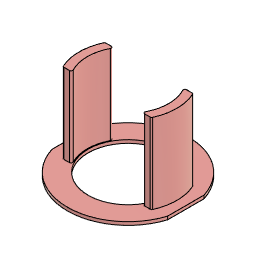
pelican TSA key retainer v1 (Autodesk Fusion 360 design; units mm, degrees)
Autodesk Fusion 360 part; units mm, degrees
note: some values were not read from the file. Set by a fixed rule: which sketch regions a step uses.
sketch "Sketch1" plane through (0, 0, 0) normal (0, 0, 1) x (1, 0, 0)
  circle A0 centre (0, 0) radius 6.3
  circle A1 centre (0, 0) radius 7.6
  line L0 (0, 7.6) -> (0, -7.6) construction
  circle A2 centre (0, 0) radius 3.25
  line L1 (-3.25, 0) -> (-3.25, -3.35)
  line L2 (-3.25, -3.35) -> (3.25, -3.35)
  line L3 (3.25, 0) -> (3.25, -3.35)
  circle A3 centre (0, 0) radius 5
  dimension "d1" = 12.6
  dimension "d2" = 15.2
  dimension "d3" = 6.5
  dimension "d4" = 3.35
  dimension "d15" = 10
  constraint coincident A0.centre A1.centre
  constraint coincident A1 L0.start
  constraint coincident A1 L0.end
  constraint vertical L0
  constraint coincident L0 A0.centre
  constraint coincident A2 L1.start
  constraint tangent A2 L1
  constraint parallel L0 L1
  constraint perpendicular L1 L2
  constraint coincident A2 L3.start
  constraint tangent A2 L3
  constraint perpendicular L2 L3
  constraint concentric A1 A3
  measures "d1" diameter of A0
  measures "d2" diameter of A1
  measures "d3" diameter of A2
  measures "d4" distance of A0.centre L2
  measures "d15" diameter of A3
extrude "Extrude1" add sketch "Sketch1" along normal blind 0.4 contours A0 | A1
sketch "Sketch2" plane through (0, 0, 0.4) normal (0, 0, 1) x (-1, 0, 0)
  circle A0 centre (0, 0) radius 7.6
  circle A1 centre (0, 0) radius 6.125
  circle A2 centre (0, 0) radius 5.1
  line L0 (-10, -2.625) -> (10, -2.625)
  line L1 (10, -2.625) -> (10, 2.625)
  line L2 (10, 2.625) -> (-10, 2.625)
  line L3 (-10, 2.625) -> (-10, -2.625)
  line L4 (-10, -2.625) -> (10, 2.625) construction
  line L5 (10, -2.625) -> (-10, 2.625) construction
  circle A3 centre (0, 0) radius 5
  dimension "d7" = 12.25
  dimension "d8" = 10.2
  dimension "d9" = 5.25
  dimension "d10" = 20
  constraint concentric A1 A2
  constraint horizontal L0
  constraint perpendicular L0 L1
  constraint parallel L0 L2
  constraint parallel L1 L3
  constraint coincident L4 A0.centre
  constraint coincident L5 A0.centre
  constraint coincident A0.centre A1.centre
  measures "d7" diameter of A1
  measures "d8" diameter of A2
  measures "d9" distance of L0.end L1.end
  measures "d10" distance of L1 L3
extrude "Extrude2" add sketch "Sketch2" along normal blind 10 contours A1 A2 L0 L2 | A1 A2 L0 L2
fillet "Fillet1" radius 0.2 8 edges at (4.3726, -2.625, 5.4) (4.3726, 2.625, 5.4) (5.534, 2.625, 5.4) (5.534, -2.625, 5.4) (-4.3726, -2.625, 5.4) (-4.3726, 2.625, 5.4) (-5.534, 2.625, 5.4) (-5.534, -2.625, 5.4)
sketch "Sketch3" plane through (0, 0, 0) normal (0, 0, -1) x (1, 0, 0)
  circle A0 centre (0, 0) radius 5
  circle A1 centre (0, 0) radius 7.6
  line L0 (-7.25, 10) -> (7.25, 10)
  line L1 (7.25, 10) -> (7.25, -10)
  line L2 (7.25, -10) -> (-7.25, -10)
  line L3 (-7.25, -10) -> (-7.25, 10)
  line L4 (-7.25, 10) -> (7.25, -10) construction
  line L5 (7.25, 10) -> (-7.25, -10) construction
  dimension "d16" = 14.5
  dimension "d17" = 20
  constraint horizontal L0
  constraint perpendicular L0 L1
  constraint parallel L0 L2
  constraint parallel L1 L3
  constraint coincident L4 A0.centre
  constraint coincident L5 A0.centre
  constraint coincident A0.centre A1.centre
  measures "d16" distance of L1.end L2.end
  measures "d17" distance of L0.end L1.end
extrude "Extrude3" cut sketch "Sketch3" against normal blind 12 contours A1 L1 | A1 L3
equation "d4 = 6.6 mm - ( d3 / 2 )"
